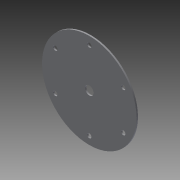
# Autodesk Inventor part: wheel_adapter
Saved by Autodesk Inventor 2014 SP1 (Build 180222100, 222)
## iProperties
Created: 2014-09-21
Part Number: wheel_adapter
Material: Générique
Document SubType Name: Modeling
Designer: astralien3000
Density: 1 g/cm^3
Appearance: Par défaut
d0: 65,000 mm
d1: 1,000 mm
d2: 0,00 deg
d3: 6,000 mm
d5: 0,00 deg
d6: 27,000 mm
d7: 3,000 mm
d8: 6,000 nd
d13: 0,00 deg
d10: 360,00 deg
Author: astralien3000
Autodesk Inventor part; units mm, degrees
ref_plane "YZ Plane" through (0, 0, 0) normal (1, 0, 0) x (0, 1, 0)
ref_plane "XZ Plane" through (0, 0, 0) normal (0, 1, 0) x (-1, 0, 0)
ref_plane "XY Plane" through (0, 0, 0) normal (0, 0, 1) x (1, 0, 0)
sketch "Esquisse1" plane through (0, 0, 0) normal (0, 1, 0) x (-1, 0, 0)
  circle A0 centre (0, 0) radius 32.5
  dimension "d0" = 65
  constraints: 1 centre point, 1 coincident
  measures "d0" diameter of A0
extrude "Extrusion1" add sketch "Esquisse1" along normal blind 1
sketch "Esquisse2" plane through (0, 1, 0) normal (0, 1, 0) x (1, 0, 0)
  circle A0 centre (0, 0) radius 32.5 projected
  circle A1 centre (0, 0) radius 3
  dimension "d3" = 6
  constraints: 1 centre point, 1 coincident
  measures "d3" diameter of A1
extrude "Extrusion2" cut sketch "Esquisse2" against normal through all contours A1
sketch "Esquisse3" plane through (0, 1, 0) normal (0, 1, 0) x (1, 0, 0)
  circle A0 centre (0, 0) radius 3 projected
  circle A1 centre (0, 0) radius 32.5 projected
  line L0 (0, 0) -> (0, 32.5) construction
  circle A2 centre (0, 27) radius 1.5
  circle A3 centre (-23.3827, 13.5) radius 1.5
  circle A4 centre (-23.3827, -13.5) radius 1.5
  circle A5 centre (0, -27) radius 1.5
  circle A6 centre (23.3827, -13.5) radius 1.5
  circle A7 centre (23.3827, 13.5) radius 1.5
  dimension "d6" = 27
  dimension "d7" = 3
  dimension "d10" = 360
  constraints: 6 centre point, 2 end point, 1 point on line, 1 vertical, 1 vertical alignment, 14 other
  measures "d6" distance of A2.centre A0.centre
  measures "d7" diameter of A2
extrude "Extrusion3" cut sketch "Esquisse3" against normal through all contours A2 | A3 | A4 | A5 | A6 | A7
